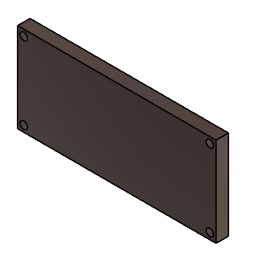
Pantalla (Autodesk Fusion 360 design; units mm, degrees)
Autodesk Fusion 360 part; units mm, degrees
sketch "Boceto2" plane through (0, 0, 0) normal (0, 1, 0) x (1, 0, 0)
  line L0 (40, 18) -> (-40, 18)
  line L1 (-40, 18) -> (-40, -18)
  line L2 (-40, -18) -> (40, -18)
  line L3 (40, -18) -> (40, 18)
  line L4 (40, 18) -> (-40, -18) construction
  line L5 (-40, 18) -> (40, -18) construction
  line L6 (37.5, 15.5) -> (-37.5, 15.5)
  line L7 (-37.5, 15.5) -> (-37.5, -15.5)
  line L8 (-37.5, -15.5) -> (37.5, -15.5)
  line L9 (37.5, -15.5) -> (37.5, 15.5)
  line L10 (37.5, 15.5) -> (-37.5, -15.5) construction
  line L11 (-37.5, 15.5) -> (37.5, -15.5) construction
  circle A0 centre (37.5, -15.5) radius 1.5
  circle A1 centre (-37.5, 15.5) radius 1.5
  circle A2 centre (-37.5, -15.5) radius 1.5
  circle A3 centre (37.5, 15.5) radius 1.5
  line L12 (26.2327, 12.7061) -> (-26.2327, 12.7061)
  line L13 (-26.2327, 12.7061) -> (-26.2327, -12.7061)
  line L14 (-26.2327, -12.7061) -> (26.2327, -12.7061)
  line L15 (26.2327, -12.7061) -> (26.2327, 12.7061)
  line L16 (26.2327, 12.7061) -> (-26.2327, -12.7061) construction
  line L17 (-26.2327, 12.7061) -> (26.2327, -12.7061) construction
  dimension "d5" = 75
  dimension "d6" = 31
  dimension "d7" = 80
  dimension "d8" = 36
  dimension "d9" = 3
  constraint horizontal L0
  constraint perpendicular L0 L1
  constraint parallel L0 L2
  constraint parallel L1 L3
  constraint coincident L4 origin
  constraint coincident L5 origin
  constraint horizontal L6
  constraint perpendicular L6 L7
  constraint parallel L6 L8
  constraint parallel L7 L9
  constraint coincident L10 origin
  constraint coincident L11 origin
  constraint equal A0 A1
  constraint equal A1 A2
  constraint equal A2 A3
  constraint coincident L8.end L9.start
  constraint coincident L6.start L9.end
  constraint coincident L7 L8.start
  constraint coincident L7.end L8.start
  constraint coincident L6.end L7.start
  constraint horizontal L12
  constraint perpendicular L12 L13
  constraint parallel L12 L14
  constraint parallel L13 L15
  constraint coincident L16 origin
  constraint coincident L17 origin
  measures "d5" distance of L7.end L8.end
  measures "d6" distance of L6.start L8.end
  measures "d7" distance of L1.end L2.end
  measures "d8" distance of L0.start L2.end
  measures "d9" diameter of A1
extrude "Extruir1" add sketch "Boceto2" along normal blind 5 contours L0 L1 L2 L3 | L6 L7 L8 L9 A0 A1 A2 A3 | L12 L13 L14 L15 makes body 1
extrude "Extruir2" add sketch "Boceto2" along normal blind 4 from surface at 5 separate body contours L12 L13 L14 L15 makes body 2
